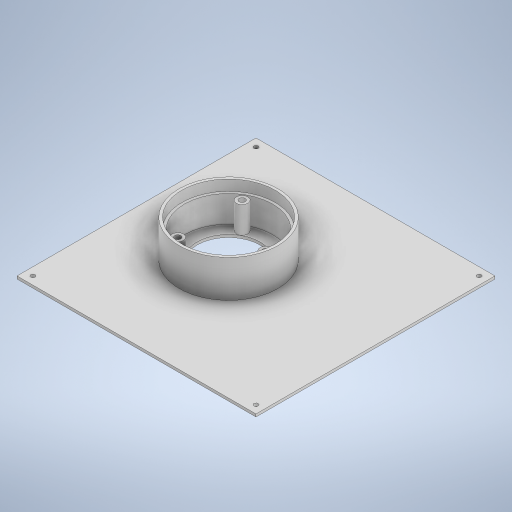
# Autodesk Inventor part: top plate
Saved by Autodesk Inventor 2024.1 (Build 281209000, 209)
## iProperties
Created: 2025-03-26
Part Number: top plate
Material: Generic
Document SubType Name: Modeling
Designer: User
Density: 1 g/cm^3
Appearance: Default
Author: User
Autodesk Inventor part; units mm, degrees
ref_plane "YZ Plane" through (0, 0, 0) normal (1, 0, 0) x (0, 1, 0)
ref_plane "XZ Plane" through (0, 0, 0) normal (0, 1, 0) x (-1, 0, 0)
ref_plane "XY Plane" through (0, 0, 0) normal (0, 0, 1) x (1, 0, 0)
sketch "Sketch1" plane through (0, 0, 0) normal (0, 1, 0) x (-1, 0, 0)
  line L0 (0, 0) -> (180, 0)
  line L1 (180, 0) -> (180, -180)
  line L2 (180, -180) -> (0, -180)
  line L3 (0, -180) -> (0, 0)
  dimension "d0" = 180
  dimension "d1" = 180
  constraints: 8 end point, 2 parallel, 1 horizontal, 1 perpendicular
  measures "d0" distance of L1.end L2.end
  measures "d1" distance of L0.end L1.end
extrude "Extrusion1" add sketch "Sketch1" along normal blind 2
sketch "Sketch3" plane through (0, 2, 0) normal (0, 1, 0) x (1, 0, 0)
  circle A0 centre (-174, 6) radius 1.65
  circle A1 centre (-174, 174) radius 1.65
  circle A2 centre (-6, 174) radius 1.65
  circle A3 centre (-6, 6) radius 1.65
  point P0 (0, 0)
  dimension "d9" = 3.3
  dimension "d10" = 3.3
  dimension "d11" = 3.3
  dimension "d12" = 3.3
  constraints: 4 centre point
  measures "d9" diameter of A0
  measures "d10" diameter of A1
  measures "d11" diameter of A2
  measures "d12" diameter of A3
extrude "Extrusion3" cut sketch "Sketch3" against normal through all
sketch "Sketch10" plane through (0, 2, 0) normal (0, 1, 0) x (1, 0, 0)
  line L0 (0, 180) -> (-180, 180)
  circle A0 centre (-110.675, 90) radius 35.2
  circle A1 centre (-110.675, 90) radius 37.2
  circle A2 centre (-110.675, 90) radius 28 construction
  line L1 (-110.675, 90) -> (-73.475, 90) construction
  line L2 (-110.675, 90) -> (-129.275, 122.216145) construction
  line L3 (-90.675, 90) -> (-53.475, 90) construction
  line L4 (-110.675, 90) -> (-129.275, 57.783855) construction
  line L5 (-90.675, 90) -> (-53.475, 90) construction
  circle A3 centre (-124.675, 114.248711) radius 2.3
  circle A4 centre (-124.675, 114.248711) radius 4.3
  circle A5 centre (-124.675, 65.751289) radius 2.3
  circle A6 centre (-124.675, 65.751289) radius 4.3
  circle A7 centre (-82.675, 90) radius 2.3
  circle A8 centre (-82.675, 90) radius 4.3
  circle A9 centre (-110.675, 90) radius 33.2
  circle A10 centre (-110.675, 90) radius 23.7
  point P0 (0, 0)
  dimension "d68" = 70.4
  dimension "d69" = 74.4
  dimension "d70" = 56
  dimension "d71" = 120
  dimension "d72" = 120
  dimension "d73" = 4.6
  dimension "d74" = 8.6
  dimension "d75" = 4.6
  dimension "d76" = 8.6
  dimension "d77" = 4.6
  dimension "d78" = 8.6
  dimension "d79" = 66.4
  dimension "d88" = 47.4
  constraints: 11 centre point, 10 end point, 8 coincident, 6 point on circle, 3 horizontal, 2 equal length, 2 point on line
  measures "d68" diameter of A0
  measures "d69" diameter of A1
  measures "d70" diameter of A2
  measures "d71" angle of L3 L2
  measures "d72" angle of L4 L5
  measures "d73" diameter of A3
  measures "d74" diameter of A4
  measures "d75" diameter of A5
  measures "d76" diameter of A6
  measures "d77" diameter of A7
  measures "d78" diameter of A8
  measures "d79" diameter of A9
  measures "d88" diameter of A10
sketch "Sketch10 outline for Extrusion11" plane through (0, 2, 0) normal (0, 1, 0) x (1, 0, 0)
  circle A0 centre (-110.675, 90) radius 35.2
  circle A1 centre (-110.675, 90) radius 33.2
  circle A2 centre (-82.675, 90) radius 4.3
  circle A3 centre (-82.675, 90) radius 2.3
  circle A4 centre (-124.675, 65.751289) radius 4.3
  circle A5 centre (-124.675, 65.751289) radius 2.3
  circle A6 centre (-124.675, 114.248711) radius 4.3
  circle A7 centre (-124.675, 114.248711) radius 2.3
extrude "Extrusion11" add sketch "Sketch10 outline for Extrusion11" along normal blind 20
sketch "Sketch10 outline for Extrusion12" plane through (0, 2, 0) normal (0, 1, 0) x (1, 0, 0)
  circle A0 centre (-110.675, 90) radius 37.2
  circle A1 centre (-110.675, 90) radius 35.2
extrude "Extrusion12" add sketch "Sketch10 outline for Extrusion12" along normal blind 28
sketch "Sketch10 outline for Extrusion13" plane through (0, 2, 0) normal (0, 1, 0) x (1, 0, 0)
  circle A0 centre (-110.675, 90) radius 23.7
extrude "Extrusion13" cut sketch "Sketch10 outline for Extrusion13" against normal through all
sketch "Sketch10 outline for Extrusion14" plane through (0, 2, 0) normal (0, 1, 0) x (1, 0, 0)
  circle A0 centre (-124.675, 114.248711) radius 2.3
  circle A1 centre (-124.675, 65.751289) radius 2.3
  circle A2 centre (-82.675, 90) radius 2.3
extrude "Extrusion14" cut sketch "Sketch10 outline for Extrusion14" against normal through all
body "Solid1"
